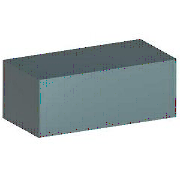
# Autodesk Inventor part: DIN 6885 - B 5 x 5 x 50
Saved by Autodesk Inventor 2025 (Build 290162000, 162)
## iProperties
Created: 2024-01-20
Part Number: DIN 6885 - B 5 x 5 x 50
Material: Steel, Mild
Description: Parallel Key
Document SubType Name: Modeling
Standard: DIN 6885-1
Designer: Abdullah
Standard Revision: 1968-08
Standards Organization: DIN
Language: en-US
Size Designation: B 5 x 5 x 50
Categories: <MemberInstance><Categories><Category DisplayName="Shaft Parts" InternalName="7f7aeb1f-a693-4053-b835-cee3144e0d98" Mnemonic="SHFT"><Category DisplayName="Keys" InternalName="7048e72f-fdca-4e3b-88b7-55969eb6630e" Mnemonic="KEY"><CategoryParameter DisplayName="Width" InternalName="34be0dd5-dba5-4911-b4ec-c22f2bfaa692" Mnemonic="kwdth"/><CategoryParameter DisplayName="Maximal Shaft Diameter" InternalName="95a81a26-4bdb-43e8-b886-6e2d08494928" Mnemonic="maxshdia"/><CategoryParameter DisplayName="Minimal Shaft Diameter" InternalName="b06394f3-cee7-4e5b-902c-663fb38acff4" Mnemonic="minshdia"/><CategoryParameter DisplayName="Key Size" InternalName="da4729c0-75a4-4053-9158-804a4a937d72" Mnemonic="keysize"/><CategoryParameter DisplayName="Shaft Diameter Range (Min.-Max.)" InternalName="e5432c95-44d4-4c4b-a96d-eed0500887aa" Mnemonic="shaftdiarng"/><CategoryParameter DisplayName="Shaft Diameter" InternalName="ff971ec2-6a20-455a-900e-83f11d6bc337" Mnemonic="shaftdia"/><Category DisplayName="Keys - Machine" InternalName="7a219f9c-bd0a-4811-91fb-2e47d97adffa" Mnemonic="PRLKEY"><CategoryParameter DisplayName="Key Type" InternalName="16552a72-3a79-47b2-9cce-0bdb5ab712ec" Mnemonic="keytype"/><CategoryParameter DisplayName="Length" InternalName="2aaf8abc-e798-4f7a-b8d4-83df963ddd80" Mnemonic="klen"/><CategoryParameter DisplayName="Parallel Key Groove Depth" InternalName="b2aecbbc-9c00-4ee8-a417-d7ce8bca5723" Mnemonic="groovedepth"/><CategoryParameter DisplayName="Height" InternalName="d0342fb0-ff3c-42cf-83d6-cbe58e85d3e8" Mnemonic="kheig"/><CategoryParameter DisplayName="Hub Depth" InternalName="e370d4da-8754-4912-963a-6e35f2b6573a" Mnemonic="hubdepth"/><Category DisplayName="Rectangular" InternalName="76fd79ae-7115-48d1-8258-5ef5a08dbe3d" Mnemonic="PRLKEYREC"/></Category></Category></Category><Category DisplayName="DataType" InternalName="23b78d0f-2648-40c6-8793-ca6db495c9e8" Mnemonic="DATATYPE"><CategoryParameter DisplayName="DisplayName" InternalName="05415f3d-3907-474b-a020-eb9d644f4cf3" Mnemonic="DISPLAYNAME"/><CategoryParameter DisplayName="Standard" InternalName="0c0a119c-1e12-4c84-803f-101930972f5e" Mnemonic="STANDARD"/><CategoryParameter DisplayName="Description" InternalName="13903e3d-64b1-4950-80da-f627842ea37f" Mnemonic="DESCRIPTION"/><CategoryParameter DisplayName="Designation" InternalName="2675968c-4ce5-49e0-a4f5-552d29089031" Mnemonic="DESIGNATION"/><CategoryParameter DisplayName="Default Row" InternalName="2af9ec52-faaa-4026-b378-f9fa4afca842" Mnemonic="DEFAULTROW"/><CategoryParameter DisplayName="Folder Name" InternalName="3f06958e-8713-4116-9be7-ed6184ecc97b" Mnemonic="FOLDERNAME"/><CategoryParameter DisplayName="Revision Guid" InternalName="45a75005-10b1-4dfc-8d6d-dfe629f0b93c" Mnemonic="REVISIONGUID"/><CategoryParameter DisplayName="FileName" InternalName="8b46a4cc-9585-4fed-90c3-899f57e09a73" Mnemonic="FILENAME"/><CategoryParameter DisplayName="StdsOrg" InternalName="8f5914e1-4693-403f-8ab5-d37768198c9d" Mnemonic="STDSORG"/><CategoryParameter DisplayName="Family Version" InternalName="914462f6-6e19-4b14-ba84-155b9680b1d0" Mnemonic="FAMILYREVISION"/><CategoryParameter DisplayName="Standard Revision" InternalName="91d5a463-65c2-4fde-b823-3b7fea5e8e17" Mnemonic="STANDARDREVISION"/><CategoryParameter DisplayName="Member Revision" InternalName="a65d44b9-392f-4f4f-857b-e4b3d54996fe" Mnemonic="MEMBERREVISION"/><CategoryParameter DisplayName="ClipFormat" InternalName="bc51e27b-3422-4e78-93ef-cec197ddf230" Mnemonic="CLIPFORMAT"/><CategoryParameter DisplayName="Manufacturer" InternalName="cd6c7a72-a28a-4e50-99a9-2c7f4e13e5ad" Mnemonic="MANUFACTURER"/><CategoryParameter DisplayName="InternalName" InternalName="cf1d0246-76d9-4b4a-8305-fa0409afb5c1" Mnemonic="INTERNALNAME"/><CategoryParameter DisplayName="IsMetric" InternalName="e2385c5b-1ea4-4823-96a8-8de651266ec3" Mnemonic="ISMETRIC"/><Category DisplayName="Part" InternalName="c0e0b642-3bcb-4cc8-9e80-f96d35c4afa4" Mnemonic="PART"><CategoryParameter DisplayName="Part Number" InternalName="016b6077-bfbe-49bd-92c9-d8d59c39c941" Mnemonic="PARTNUMBER"/><CategoryParameter DisplayName="Stock Number" InternalName="4dba7c1c-e26c-444e-836c-b08b433409a8" Mnemonic="STOCKNUMBER"/><CategoryParameter DisplayName="Material Key" InternalName="5c9a8adb-dd2b-4535-b97f-0a94a95fe41f" Mnemonic="MATERIALKEY"/><CategoryParameter DisplayName="Material" InternalName="818a152a-d3c3-49ca-80ee-df7d91421b8e" Mnemonic="MATERIAL"/></Category></Category><Category DisplayName="LegacyMap" InternalName="cd87c42b-3e48-431e-b5c0-1cbeb14dfe77" Mnemonic="LEGACYMAP"><CategoryParameter DisplayName="unique DA member ID" InternalName="0918ad47-427f-4fed-ae26-24c81c58f590" Mnemonic="DACOOKIE"/><CategoryParameter DisplayName="Merge11 ID" InternalName="0ee8fb18-e2ed-4f39-96f6-1f4b5f50aa71" Mnemonic="MERGE11"/><CategoryParameter DisplayName="unique CC member ID" InternalName="5193edd4-b2b0-4ab4-9d54-de900eee34e0" Mnemonic="CCCOOKIE"/><CategoryParameter DisplayName="Split ID" InternalName="72b5c83c-be7f-45c4-ae51-9160ea6deb26" Mnemonic="SPLIT"/><CategoryParameter DisplayName="MemberID" InternalName="8e5e0294-fc51-4c8f-b3d7-003dc5ed94f6" Mnemonic="MEMBERID"/><CategoryParameter DisplayName="CatalogName" InternalName="d99d1e27-aa94-4de2-af4c-c348882a6f4f" Mnemonic="CATALOGNAME"/><CategoryParameter DisplayName="FamilyNumber" InternalName="e705e1f4-09cb-413e-91f9-551b4188271e" Mnemonic="FAMILYNUMBER"/></Category></Categories><FamilyTemplate Id="si0116"><FamilyTemplateParameters><FamilyTemplateParameter ObjectType="kUserParameterObject" ValueType="xs:double" Id="1" ObjectReferenceKey="NLG"/><FamilyTemplateParameter ObjectType="kUserParameterObject" ValueType="xs:double" Id="2" ObjectReferenceKey="RR"/><FamilyTemplateParameter ObjectType="kUserParameterObject" ValueType="xs:double" Id="3" ObjectReferenceKey="WDMIN"/><FamilyTemplateParameter ObjectType="kUserParameterObject" ValueType="xs:double" Id="4" ObjectReferenceKey="PH"/><FamilyTemplateParameter ObjectType="kUserParameterObject" ValueType="xs:double" Id="5" ObjectReferenceKey="PHH"/><FamilyTemplateParameter ObjectType="kUserParameterObject" ValueType="xs:double" Id="6" ObjectReferenceKey="PNT"/><FamilyTemplateParameter ObjectType="kUserParameterObject" ValueType="xs:double" Id="7" ObjectReferenceKey="WDMAX"/><FamilyTemplateParameter ObjectType="kUserParameterObject" ValueType="xs:double" Id="8" ObjectReferenceKey="PLB1"/><FamilyTemplateParameter ObjectType="kUserParameterObject" ValueType="xs:double" Id="9" ObjectReferenceKey="PB"/><FamilyTemplateParameter ObjectType="kUserParameterObject" ValueType="xs:double" Id="10" ObjectReferenceKey="PLB2"/><FamilyTemplateParameter ObjectType="kUserParameterObject" ValueType="xs:double" Id="11" ObjectReferenceKey="PUEB"/><FamilyTemplateParameter ObjectType="kPropertyObject" ValueType="xs:string" Id="100" ObjectReferenceKey="{32853F0F-3444-11d1-9E93-0060B03C1CA6}" SubObjectId="52"/><FamilyTemplateParameter ObjectType="kPropertyObject" ValueType="xs:string" Id="105" ObjectReferenceKey="{32853F0F-3444-11d1-9E93-0060B03C1CA6}" SubObjectId="5"/><FamilyTemplateParameter ObjectType="kPartComponentDefinitionObject" ValueType="xs:string" Id="110" SubObjectId="Material"/></FamilyTemplateParameters></FamilyTemplate><CategoryParameterMap><ParamToTemplateMap><ParamToTemplate CategoryParameter="//CategoryParameter[@InternalName='05415f3d-3907-474b-a020-eb9d644f4cf3']" ConstantValue="DIN 6885-1 B"/><ParamToTemplate CategoryParameter="//CategoryParameter[@InternalName='cf1d0246-76d9-4b4a-8305-fa0409afb5c1']" ConstantValue="5b84c1cb-a235-433e-badf-de8bc13a8937"/><ParamToTemplate CategoryParameter="//CategoryParameter[@InternalName='3f06958e-8713-4116-9be7-ed6184ecc97b']" ConstantValue="DIN 6885-1 B"/><ParamToTemplate CategoryParameter="//CategoryParameter[@InternalName='914462f6-6e19-4b14-ba84-155b9680b1d0']" ConstantValue="10"/><ParamToTemplate CategoryParameter="//CategoryParameter[@InternalName='bc51e27b-3422-4e78-93ef-cec197ddf230']" ConstantValue="CF_INVENTOR.STDPARTS"/><ParamToTemplate CategoryParameter="//CategoryParameter[@InternalName='e2385c5b-1ea4-4823-96a8-8de651266ec3']" ConstantValue="true"/><ParamToTemplate CategoryParameter="//CategoryParameter[@InternalName='13903e3d-64b1-4950-80da-f627842ea37f']" ConstantValue="Parallel Key"/><ParamToTemplate CategoryParameter="//CategoryParameter[@InternalName='8f5914e1-4693-403f-8ab5-d37768198c9d']" ConstantValue="DIN"/><ParamToTemplate CategoryParameter="//CategoryParameter[@InternalName='0c0a119c-1e12-4c84-803f-101930972f5e']" ConstantValue="DIN 6885-1"/><ParamToTemplate CategoryParameter="//CategoryParameter[@InternalName='cd6c7a72-a28a-4e50-99a9-2c7f4e13e5ad']" TemplateParameter="104"/><ParamToTemplate CategoryParameter="//CategoryParameter[@InternalName='91d5a463-65c2-4fde-b823-3b7fea5e8e17']" ConstantValue="1968-08"/><ParamToTemplate CategoryParameter="//CategoryParameter[@InternalName='45a75005-10b1-4dfc-8d6d-dfe629f0b93c']" ConstantValue="b135cd93-d60e-49c9-844a-fcad66b2100c"/><ParamToTemplate CategoryParameter="//CategoryParameter[@InternalName='2af9ec52-faaa-4026-b378-f9fa4afca842']" ConstantValue="3010"/><ParamToTemplate CategoryParameter="//CategoryParameter[@InternalName='d99d1e27-aa94-4de2-af4c-c348882a6f4f']" ConstantValue="DIN"/><ParamToTemplate CategoryParameter="//CategoryParameter[@InternalName='e705e1f4-09cb-413e-91f9-551b4188271e']" ConstantValue="292"/><ParamToTemplate CategoryParameter="//CategoryParameter[@InternalName='8b46a4cc-9585-4fed-90c3-899f57e09a73']" ConstantValue="DIN 6885 - B 5 x 5 x 50"/><ParamToTemplate CategoryParameter="//CategoryParameter[@InternalName='a65d44b9-392f-4f4f-857b-e4b3d54996fe']" ConstantValue="1FF821D0-517C-4AE2-B39F-350FC8C6F41E"/><ParamToTemplate CategoryParameter="//CategoryParameter[@InternalName='e5432c95-44d4-4c4b-a96d-eed0500887aa']" ConstantValue="12 - 17"/><ParamToTemplate CategoryParameter="//CategoryParameter[@InternalName='da4729c0-75a4-4053-9158-804a4a937d72']" ConstantValue="5x5"/><ParamToTemplate CategoryParameter="//CategoryParameter[@InternalName='16552a72-3a79-47b2-9cce-0bdb5ab712ec']" ConstantValue="B"/><ParamToTemplate CategoryParameter="//CategoryParameter[@InternalName='8e5e0294-fc51-4c8f-b3d7-003dc5ed94f6']" ConstantValue="3490"/><ParamToTemplate CategoryParameter="//CategoryParameter[@InternalName='2675968c-4ce5-49e0-a4f5-552d29089031']" TemplateParameter="100"/><ParamToTemplate CategoryParameter="//CategoryParameter[@InternalName='818a152a-d3c3-49ca-80ee-df7d91421b8e']" TemplateParameter="110"/><ParamToTemplate CategoryParameter="//CategoryParameter[@InternalName='2aaf8abc-e798-4f7a-b8d4-83df963ddd80']" TemplateParameter="1"/><ParamToTemplate CategoryParameter="//CategoryParameter[@InternalName='016b6077-bfbe-49bd-92c9-d8d59c39c941']" TemplateParameter="105"/><ParamToTemplate CategoryParameter="//CategoryParameter[@InternalName='34be0dd5-dba5-4911-b4ec-c22f2bfaa692']" TemplateParameter="9"/><ParamToTemplate CategoryParameter="//CategoryParameter[@InternalName='d0342fb0-ff3c-42cf-83d6-cbe58e85d3e8']" TemplateParameter="4"/><ParamToTemplate CategoryParameter="//CategoryParameter[@InternalName='b2aecbbc-9c00-4ee8-a417-d7ce8bca5723']" TemplateParameter="6"/><ParamToTemplate CategoryParameter="//CategoryParameter[@InternalName='e370d4da-8754-4912-963a-6e35f2b6573a']" TemplateParameter="11"/><ParamToTemplate CategoryParameter="//CategoryParameter[@InternalName='95a81a26-4bdb-43e8-b886-6e2d08494928']" TemplateParameter="7"/><ParamToTemplate CategoryParameter="//CategoryParameter[@InternalName='b06394f3-cee7-4e5b-902c-663fb38acff4']" TemplateParameter="3"/></ParamToTemplateMap></CategoryParameterMap></MemberInstance>
Density: 7.85 g/cm^3
Appearance: Semi-Polished
IsCustomPart: 0
Author: Abdullah
Autodesk Inventor part; units mm, degrees
ref_plane "YZ Plane" through (0, 0, 0) normal (1, 0, 0) x (0, 1, 0)
sketch "Sketch1" plane through (0, 0, 0) normal (0, 0, 1) x (1, 0, 0)
  line L0 (2.5, 2.5) -> (52.5, 2.5)
  line L1 (52.5, 2.5) -> (52.5, -2.5)
  line L2 (52.5, -2.5) -> (2.5, -2.5)
  arc A0 (2.5, 2.5) -> (2.5, -2.5) centre (2.5, 0) ccw construction
  line L3 (0, 7) -> (0, -7) projected
  line L4 (-6, 0) -> (36, 0) projected
  line L5 (2.5, 2.5) -> (2.5, -2.5)
  dimension "d0" = 2.5
  dimension "d13" = 50
  constraints: 8 end point, 3 tangent, 2 perpendicular, 2 point on circle, 1 centre point, 1 horizontal, 1 parallel, 1 point on line
  measures "d0" radius of A0
  measures "d13" distance between parallel lines of L1 L5
ref_plane "Work Plane1" through (0, 0, -3) normal (0, 0, 1) x (1, 0, 0)
ref_plane "Work Plane2" through (0, 0, 2) normal (0, 0, 1) x (1, 0, 0)
extrude "Body1" add sketch "Sketch1" against normal up to surface (5 mm away) from surface at 2
equation "\"d0\" = 0.5 * PB"
equation "\"d13\" = NLG"
equation "\"d1\" = -PNT"
equation "\"d2\" = PH - PNT"
equation "\"NLG\" = 50"
equation "\"PB\" = 5"
equation "\"PNT\" = 3"
equation "\"PH\" = 5"
equation "\"PHH\" = 0"
equation "\"RR\" = 0.001"
equation "\"WDMIN\" = 12"
equation "\"WDMAX\" = 17"
equation "\"PLB1\" = 52.5"
equation "\"PLB2\" = 55"
equation "\"PUEB\" = 2.3"
body "Solid1"
